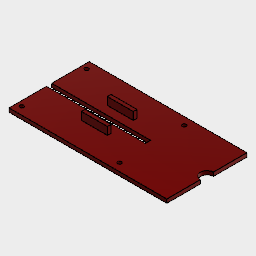
AnimationFrame v30 (Autodesk Fusion 360 design; units mm, degrees)
Autodesk Fusion 360 part; units mm, degrees
sketch "Sketch1" plane through (0, 0, 0) normal (0, 1, 0) x (1, 0, 0)
  line L0 (0, 0) -> (122, 0)
  line L1 (122, 0) -> (122, -62)
  line L2 (122, -62) -> (0, -62)
  line L3 (0, -62) -> (0, 0)
  dimension "d1" = 122
  dimension "d2" = 62
  constraint horizontal L0
  constraint vertical L1
  constraint horizontal L2
  constraint vertical L3
  constraint coincident L0.start L3.end
  measures "d2" distance of L0.start
extrude "Extrude1" add sketch "Sketch1" along normal blind 3
sketch "Sketch2" plane through (0, 3, 0) normal (0, 1, 0) x (-1, 0, 0)
  line L0 (0, 62) -> (-122, 62)
  line L1 (-122, 62) -> (-122, 0)
  line L2 (-122, 0) -> (0, 0)
  line L3 (0, 0) -> (0, 62)
  line L4 (0, 31) -> (-122, 31) construction
  line L5 (0, 29) -> (-76.5, 29)
  line L6 (-76.5, 29) -> (-76.5, 33)
  line L7 (-76.5, 33) -> (0, 33)
  line L8 (0, 33) -> (0, 29)
  line L9 (-76.5, 22.4) -> (0, 22.4)
  line L10 (0, 22.4) -> (0, 19.6)
  line L11 (0, 19.6) -> (-76.5, 19.6)
  line L12 (-76.5, 19.6) -> (-76.5, 22.4)
  line L13 (-76.5, 21) -> (0, 21) construction
  line L14 (-76.5, 39.6) -> (0, 39.6)
  line L15 (0, 39.6) -> (0, 42.4)
  line L16 (0, 42.4) -> (-76.5, 42.4)
  line L17 (-76.5, 42.4) -> (-76.5, 39.6)
  line L18 (0, 41) -> (-76.5, 41) construction
  circle A0 centre (-74, 31) radius 2 construction
  line L19 (-76.5, 10) -> (-76.5, 55) construction
  line L20 (-36.5, 10) -> (-36.5, 51)
  dimension "d22" = 4
  dimension "d25" = 2.8
  dimension "d26" = 2.8
  dimension "d27" = 10
  dimension "d28" = 10
  dimension "d29" = 2.5
  dimension "d30" = 76.5
  dimension "d33" = 2
  dimension "d34" = 40
  constraint midpoint L3
  constraint midpoint L1
  constraint horizontal L5
  constraint vertical L6
  constraint horizontal L7
  constraint vertical L8
  constraint collinear L3 L8
  constraint horizontal L9
  constraint vertical L10
  constraint horizontal L11
  constraint vertical L12
  constraint coincident L3
  constraint midpoint L12
  constraint midpoint L10
  constraint horizontal L14
  constraint vertical L15
  constraint horizontal L16
  constraint vertical L17
  constraint midpoint L15
  constraint midpoint L17
  constraint coincident L4
  constraint tangent L5 A0
  constraint vertical L19
  constraint collinear L12 L19
  constraint collinear L17 L19
  constraint collinear L6 L19
  constraint perpendicular L13 L20
  measures "d22" distance of L2.end
  measures "d26" distance of L2.end
  measures "d27" distance of L4 L18
  measures "d28" distance of L4 L13
  measures "d29" distance of L6
  measures "d30" distance of L3 L19
  measures "d33" distance of L4 L5
  measures "d34" distance of L19 L20
extrude "Extrude2" cut sketch "Sketch2" against normal through all contours L3 L5 L7 L8 L20 | L5 L6 L7 L20
sketch "Sketch3" plane through (0, 3, 0) normal (0, 1, 0) x (-1, 0, 0)
  line L0 (0, 62) -> (-122, 62)
  line L1 (-122, 62) -> (-122, 0)
  line L2 (-122, 0) -> (0, 0)
  line L3 (0, 33) -> (0, 62)
  circle A0 centre (-122, 31) radius 5
  line L4 (0, 29) -> (-76.5, 29)
  line L5 (-76.5, 29) -> (-76.5, 33)
  line L6 (-76.5, 33) -> (0, 33)
  line L7 (0, 0) -> (0, 29)
  dimension "d11" = 10
  constraint midpoint L1
  measures "d11" diameter of A0
extrude "Extrude3" cut sketch "Sketch3" against normal through all contours L1 A0 picked at (-119.9313, 30.4629)
extrude "Extrude5" add sketch "Sketch2" along normal blind 6 contours L14 L16 L17 L20 | L9 L11 L12 L20
sketch "Sketch5" plane through (0, 3, 0) normal (0, 1, 0) x (-1, 0, 0)
  line L0 (-76.5, 39.6) -> (-76.5, 42.4)
  line L1 (-76.5, 42.4) -> (-36.5, 42.4)
  line L2 (-36.5, 42.4) -> (-36.5, 39.6)
  line L3 (-36.5, 39.6) -> (-76.5, 39.6)
  line L4 (-36.5, 19.6) -> (-76.5, 19.6)
  line L5 (-76.5, 19.6) -> (-76.5, 22.4)
  line L6 (-76.5, 22.4) -> (-36.5, 22.4)
  line L7 (-36.5, 22.4) -> (-36.5, 19.6)
  arc A0 (-122, 26) -> (-122, 36) centre (-122, 31) ccw
  line L8 (-122, 26) -> (-122, 0)
  line L9 (-122, 0) -> (0, 0)
  line L10 (0, 0) -> (0, 29)
  line L11 (0, 29) -> (-76.5, 29)
  line L12 (-76.5, 29) -> (-76.5, 33)
  line L13 (-76.5, 33) -> (0, 33)
  line L14 (0, 33) -> (0, 62)
  line L15 (0, 62) -> (-122, 62)
  line L16 (-122, 62) -> (-122, 36)
  line L17 (-4, -5) -> (-4, 85) construction
  circle A1 centre (-4, 56) radius 1.5
  circle A2 centre (-4, 6) radius 1.5
  line L18 (-76.5, 31) -> (13, 31) construction
  line L19 (-79.5, -4) -> (-79.5, 69) construction
  line L20 (36.5051, 56) -> (-130, 56) construction
  circle A3 centre (-79.5, 56) radius 1.5
  circle A4 centre (-79.5, 6) radius 1.5
  dimension "d35" = 4
  dimension "d36" = 25
  dimension "d37" = 25
  dimension "d38" = 3
  dimension "d39" = 3
  dimension "d41" = 42.5
  dimension "d42" = 3
  dimension "d43" = 3
  constraint vertical L17
  constraint coincident L17
  constraint coincident L17 L9.end
  constraint midpoint L12
  constraint perpendicular L12 L18
  constraint perpendicular L15 L19
  constraint perpendicular L17 L20
  constraint coincident L19
  constraint coincident L20
  constraint coincident L19 L9.end
  measures "d35" distance of L14 L17
  measures "d36" distance of L9.end L18
  measures "d37" distance of L18
  measures "d38" diameter of A1
  measures "d39" diameter of A2
  measures "d41" distance of L8 L19
  measures "d42" diameter of A4
  measures "d43" diameter of A3
extrude "Extrude6" cut sketch "Sketch5" against normal through all contours A1 | A2 | A3 | A4
sketch "Sketch6" plane through (0, 9, 0) normal (0, 1, 0) x (-1, 0, 0)
  line L0 (-76.5, 39.6) -> (-36.5, 39.6)
  line L1 (-36.5, 39.6) -> (-36.5, 42.4)
  line L2 (-36.5, 42.4) -> (-76.5, 42.4)
  line L3 (-76.5, 42.4) -> (-76.5, 39.6)
  line L4 (-76.5, 19.6) -> (-56.5, 19.6)
  line L5 (-56.5, 19.6) -> (-56.5, 42.4)
  line L6 (-56.5, 42.4) -> (-76.5, 42.4)
  line L7 (-76.5, 42.4) -> (-76.5, 19.6)
  dimension "d44" = 20
  constraint horizontal L4
  constraint vertical L5
  constraint horizontal L6
  constraint vertical L7
  constraint coincident L2
extrude "Extrude7" cut sketch "Sketch6" against normal up to surface (6 mm away) contours L0 L2 L3 L5 L6 L7 | L0 L4 L5 L7
